Autodesk Fusion 360 part; units mm, degrees
(part 2 of 2)
  spline S235 degree 3 poles (6.52, 51.4668) (6.4718, 51.4632) (6.3612, 51.455) (6.2503, 51.4547) (6.1877, 51.4545) knots 0 0 0 0 0.014491 0.033263 0.033263 0.033263 0.033263
  spline S236 degree 3 poles (6.1877, 51.4545) (6.1361, 51.4547) (6.0447, 51.4549) (5.9536, 51.4611) (5.9138, 51.4637) knots 0 0 0 0 0.015463 0.027406 0.027406 0.027406 0.027406
  spline S237 degree 3 poles (5.9138, 51.4637) (5.8835, 51.4668) (5.8299, 51.4722) (5.7791, 51.4899) (5.7569, 51.4976) knots 0 0 0 0 0.009095 0.016102 0.016102 0.016102 0.016102
  spline S238 degree 3 poles (5.7569, 51.4976) (5.7399, 51.506) (5.7078, 51.5219) (5.6847, 51.5493) (5.6738, 51.5622) knots 0 0 0 0 0.00562 0.010625 0.010625 0.010625 0.010625
  spline S239 degree 3 poles (5.6738, 51.5622) (5.6645, 51.5771) (5.6442, 51.6095) (5.6295, 51.6447) (5.6215, 51.6637) knots 0 0 0 0 0.005277 0.011439 0.011439 0.011439 0.011439
  line L59 (5.6215, 51.6637) -> (3.3385, 58.3653)
  line L60 (3.3385, 58.3653) -> (3.3323, 58.3653)
  line L61 (3.3323, 58.3653) -> (1.1108, 51.676)
  spline S240 degree 3 poles (1.1108, 51.676) (1.1048, 51.6553) (1.0938, 51.617) (1.0759, 51.5815) (1.0677, 51.5653) knots 0 0 0 0 0.006471 0.011908 0.011908 0.011908 0.011908
  spline S241 degree 3 poles (1.0677, 51.5653) (1.0572, 51.5514) (1.0346, 51.5214) (1.0001, 51.5059) (0.9815, 51.4976) knots 0 0 0 0 0.005123 0.011115 0.011115 0.011115 0.011115
  spline S242 degree 3 poles (0.9815, 51.4976) (0.9571, 51.4899) (0.901, 51.4722) (0.8423, 51.4668) (0.8092, 51.4637) knots 0 0 0 0 0.007671 0.017604 0.017604 0.017604 0.017604
  spline S243 degree 3 poles (0.8092, 51.4637) (0.7662, 51.4611) (0.6678, 51.4549) (0.5693, 51.4547) (0.5138, 51.4545) knots 0 0 0 0 0.012942 0.029559 0.029559 0.029559 0.029559
  spline S244 degree 3 poles (0.5138, 51.4545) (0.4569, 51.4547) (0.3561, 51.4551) (0.2559, 51.4654) (0.2123, 51.4699) knots 0 0 0 0 0.017081 0.030209 0.030209 0.030209 0.030209
  spline S245 degree 3 poles (0.2123, 51.4699) (0.1801, 51.4746) (0.125, 51.4825) (0.0802, 51.5149) (0.0615, 51.5284) knots 0 0 0 0 0.009571 0.01638 0.01638 0.01638 0.01638
  spline S246 degree 3 poles (0.0615, 51.5284) (0.0504, 51.5455) (0.0257, 51.5837) (0.029, 51.6294) (0.0308, 51.6545) knots 0 0 0 0 0.005987 0.013301 0.013301 0.013301 0.013301
  spline S247 degree 3 poles (0.0308, 51.6545) (0.0364, 51.6868) (0.0494, 51.7613) (0.0748, 51.8325) (0.0892, 51.873) knots 0 0 0 0 0.009806 0.02265 0.02265 0.02265 0.02265
  line L62 (0.0892, 51.873) -> (2.6862, 59.2699)
  spline S248 degree 3 poles (-5.6769, 59.0176) (-5.6766, 59.0522) (-5.6759, 59.1171) (-5.6682, 59.1815) (-5.6646, 59.2114) knots 0 0 0 0 0.010389 0.019436 0.019436 0.019436 0.019436
  spline S249 degree 3 poles (-5.6646, 59.2114) (-5.6602, 59.2372) (-5.6518, 59.2853) (-5.6311, 59.3294) (-5.6215, 59.3499) knots 0 0 0 0 0.007801 0.014559 0.014559 0.014559 0.014559
  spline S250 degree 3 poles (-5.6215, 59.3499) (-5.6115, 59.3667) (-5.5929, 59.3978) (-5.5641, 59.4198) (-5.5508, 59.4299) knots 0 0 0 0 0.005804 0.010768 0.010768 0.010768 0.010768
  spline S251 degree 3 poles (-5.5508, 59.4299) (-5.537, 59.4371) (-5.509, 59.4516) (-5.4775, 59.4535) (-5.4615, 59.4545) knots 0 0 0 0 0.004616 0.009349 0.009349 0.009349 0.009349
  line L63 (-5.4615, 59.4545) -> (-1.64, 59.4545)
  spline S252 degree 3 poles (-1.64, 59.4545) (-1.5929, 59.4501) (-1.4957, 59.4409) (-1.4143, 59.3869) (-1.3723, 59.3591) knots 0 0 0 0 0.013974 0.028812 0.028812 0.028812 0.028812
  spline S253 degree 3 poles (-1.3723, 59.3591) (-1.3356, 59.3174) (-1.2523, 59.2225) (-1.2484, 59.0951) (-1.2462, 59.0237) knots 0 0 0 0 0.016203 0.03683 0.03683 0.03683 0.03683
  line L64 (-1.2462, 59.0237) -> (-1.2462, 51.9222)
  spline S254 degree 3 poles (-1.2462, 51.9222) (-1.2484, 51.8509) (-1.2523, 51.7235) (-1.3356, 51.6286) (-1.3723, 51.5868) knots 0 0 0 0 0.020627 0.03683 0.03683 0.03683 0.03683
  spline S255 degree 3 poles (-1.3723, 51.5868) (-1.4143, 51.559) (-1.4957, 51.505) (-1.5929, 51.4959) (-1.64, 51.4914) knots 0 0 0 0 0.014838 0.028813 0.028813 0.028813 0.028813
  line L65 (-1.64, 51.4914) -> (-5.4185, 51.4914)
  spline S256 degree 3 poles (-5.4185, 51.4914) (-5.4344, 51.4924) (-5.4659, 51.4943) (-5.4939, 51.5089) (-5.5077, 51.516) knots 0 0 0 0 0.004732 0.009349 0.009349 0.009349 0.009349
  spline S257 degree 3 poles (-5.5077, 51.516) (-5.5206, 51.5261) (-5.5484, 51.5476) (-5.564, 51.5792) (-5.5723, 51.596) knots 0 0 0 0 0.004849 0.010403 0.010403 0.010403 0.010403
  spline S258 degree 3 poles (-5.5723, 51.596) (-5.5803, 51.6167) (-5.5977, 51.6616) (-5.6072, 51.7089) (-5.6123, 51.7345) knots 0 0 0 0 0.006618 0.014436 0.014436 0.014436 0.014436
  spline S259 degree 3 poles (-5.6123, 51.7345) (-5.6168, 51.7655) (-5.6267, 51.8338) (-5.6273, 51.9029) (-5.6277, 51.9407) knots 0 0 0 0 0.009379 0.020693 0.020693 0.020693 0.020693
  spline S260 degree 3 poles (-5.6277, 51.9407) (-5.6272, 51.9753) (-5.6264, 52.0403) (-5.6168, 52.1046) (-5.6123, 52.1345) knots 0 0 0 0 0.010392 0.019465 0.019465 0.019465 0.019465
  spline S261 degree 3 poles (-5.6123, 52.1345) (-5.6073, 52.1599) (-5.598, 52.2063) (-5.5803, 52.2501) (-5.5723, 52.2699) knots 0 0 0 0 0.007743 0.014145 0.014145 0.014145 0.014145
  spline S262 degree 3 poles (-5.5723, 52.2699) (-5.5639, 52.2859) (-5.5479, 52.3163) (-5.5206, 52.337) (-5.5077, 52.3468) knots 0 0 0 0 0.005357 0.010155 0.010155 0.010155 0.010155
  spline S263 degree 3 poles (-5.5077, 52.3468) (-5.4939, 52.354) (-5.4659, 52.3685) (-5.4344, 52.3705) (-5.4185, 52.3714) knots 0 0 0 0 0.004616 0.009349 0.009349 0.009349 0.009349
  line L66 (-5.4185, 52.3714) -> (-2.3046, 52.3714)
  line L67 (-2.3046, 52.3714) -> (-2.3046, 54.8699)
  line L68 (-2.3046, 54.8699) -> (-4.9754, 54.8699)
  spline S264 degree 3 poles (-4.9754, 54.8699) (-4.9914, 54.871) (-5.0233, 54.8733) (-5.0509, 54.8895) (-5.0646, 54.8976) knots 0 0 0 0 0.004743 0.009456 0.009456 0.009456 0.009456
  spline S265 degree 3 poles (-5.0646, 54.8976) (-5.0776, 54.908) (-5.1046, 54.9297) (-5.1228, 54.9592) (-5.1323, 54.9745) knots 0 0 0 0 0.004957 0.010314 0.010314 0.010314 0.010314
  spline S266 degree 3 poles (-5.1323, 54.9745) (-5.1411, 54.9938) (-5.1607, 55.0369) (-5.1682, 55.0839) (-5.1723, 55.1099) knots 0 0 0 0 0.006314 0.014174 0.014174 0.014174 0.014174
  spline S267 degree 3 poles (-5.1723, 55.1099) (-5.1759, 55.1411) (-5.1836, 55.2086) (-5.1843, 55.2765) (-5.1846, 55.313) knots 0 0 0 0 0.00943 0.020357 0.020357 0.020357 0.020357
  spline S268 degree 3 poles (-5.1846, 55.313) (-5.1843, 55.3474) (-5.1837, 55.4112) (-5.1759, 55.4745) (-5.1723, 55.5037) knots 0 0 0 0 0.010312 0.01913 0.01913 0.01913 0.01913
  spline S269 degree 3 poles (-5.1723, 55.5037) (-5.1681, 55.5282) (-5.1603, 55.573) (-5.141, 55.6142) (-5.1323, 55.633) knots 0 0 0 0 0.007409 0.013581 0.013581 0.013581 0.013581
  spline S270 degree 3 poles (-5.1323, 55.633) (-5.123, 55.648) (-5.1054, 55.6764) (-5.0777, 55.695) (-5.0646, 55.7037) knots 0 0 0 0 0.005231 0.009893 0.009893 0.009893 0.009893
  spline S271 degree 3 poles (-5.0646, 55.7037) (-5.0507, 55.71) (-5.0224, 55.7229) (-4.9913, 55.7245) (-4.9754, 55.7253) knots 0 0 0 0 0.004529 0.009252 0.009252 0.009252 0.009252
  line L69 (-4.9754, 55.7253) -> (-2.3046, 55.7253)
  line L70 (-2.3046, 55.7253) -> (-2.3046, 58.5745)
  line L71 (-2.3046, 58.5745) -> (-5.4615, 58.5745)
  spline S272 degree 3 poles (-5.4615, 58.5745) (-5.4775, 58.5755) (-5.509, 58.5774) (-5.537, 58.5919) (-5.5508, 58.5991) knots 0 0 0 0 0.004732 0.009348 0.009348 0.009348 0.009348
  spline S273 degree 3 poles (-5.5508, 58.5991) (-5.564, 58.609) (-5.5924, 58.6302) (-5.6114, 58.6601) (-5.6215, 58.676) knots 0 0 0 0 0.004915 0.010531 0.010531 0.010531 0.010531
  spline S274 degree 3 poles (-5.6215, 58.676) (-5.6312, 58.6958) (-5.6521, 58.7387) (-5.6602, 58.7859) (-5.6646, 58.8114) knots 0 0 0 0 0.006545 0.014271 0.014271 0.014271 0.014271
  spline S275 degree 3 poles (-5.6646, 58.8114) (-5.6682, 58.8424) (-5.6761, 58.9109) (-5.6766, 58.9798) (-5.6769, 59.0176) knots 0 0 0 0 0.009353 0.020665 0.020665 0.020665 0.020665
  spline S276 degree 3 poles (-13.4185, 59.0176) (-13.4172, 59.056) (-13.4149, 59.1281) (-13.3892, 59.1954) (-13.3771, 59.2268) knots 0 0 0 0 0.011431 0.021461 0.021461 0.021461 0.021461
  spline S277 degree 3 poles (-13.3771, 59.2268) (-13.3626, 59.254) (-13.3342, 59.3071) (-13.2903, 59.3483) (-13.2689, 59.3684) knots 0 0 0 0 0.009183 0.01792 0.01792 0.01792 0.01792
  spline S278 degree 3 poles (-13.2689, 59.3684) (-13.246, 59.3855) (-13.2003, 59.4198) (-13.1463, 59.4389) (-13.1194, 59.4484) knots 0 0 0 0 0.008537 0.01705 0.01705 0.01705 0.01705
  spline S279 degree 3 poles (-13.1194, 59.4484) (-13.0919, 59.4555) (-13.0377, 59.4697) (-12.9816, 59.4719) (-12.9538, 59.473) knots 0 0 0 0 0.008479 0.016779 0.016779 0.016779 0.016779
  line L72 (-12.9538, 59.473) -> (-12.6038, 59.473)
  spline S280 degree 3 poles (-12.6038, 59.473) (-12.5519, 59.472) (-12.4542, 59.47) (-12.3589, 59.449) (-12.3142, 59.4391) knots 0 0 0 0 0.015537 0.029222 0.029222 0.029222 0.029222
  spline S281 degree 3 poles (-12.3142, 59.4391) (-12.2729, 59.4252) (-12.188, 59.3965) (-12.1158, 59.3433) (-12.0788, 59.316) knots 0 0 0 0 0.013 0.026713 0.026713 0.026713 0.026713
  spline S282 degree 3 poles (-12.0788, 59.316) (-12.0405, 59.282) (-11.958, 59.2086) (-11.8916, 59.1203) (-11.856, 59.073) knots 0 0 0 0 0.015332 0.033042 0.033042 0.033042 0.033042
  spline S283 degree 3 poles (-11.856, 59.073) (-11.8168, 59.0151) (-11.7307, 58.8882) (-11.6588, 58.7528) (-11.6196, 58.6791) knots 0 0 0 0 0.020961 0.045964 0.045964 0.045964 0.045964
  line L73 (-11.6196, 58.6791) -> (-9.1904, 54.1499)
  spline S284 degree 3 poles (-9.1904, 54.1499) (-9.1262, 54.0304) (-8.9953, 53.7868) (-8.8701, 53.5402) (-8.8064, 53.4145) knots 0 0 0 0 0.040696 0.082963 0.082963 0.082963 0.082963
  spline S285 degree 3 poles (-8.8064, 53.4145) (-8.7435, 53.2884) (-8.6202, 53.0407) (-8.5034, 52.7899) (-8.4462, 52.6668) knots 0 0 0 0 0.042275 0.082998 0.082998 0.082998 0.082998
  line L74 (-8.4462, 52.6668) -> (-8.4338, 52.6668)
  spline S286 degree 3 poles (-8.4338, 52.6668) (-8.4377, 52.816) (-8.4455, 53.1175) (-8.45, 53.4191) (-8.4523, 53.5714) knots 0 0 0 0 0.044782 0.090481 0.090481 0.090481 0.090481
  spline S287 degree 3 poles (-8.4523, 53.5714) (-8.4541, 53.7248) (-8.4577, 54.0304) (-8.4582, 54.336) (-8.4585, 54.4884) knots 0 0 0 0 0.046002 0.091695 0.091695 0.091695 0.091695
  line L75 (-8.4585, 54.4884) -> (-8.4585, 59.2945)
  spline S288 degree 3 poles (-8.4585, 59.2945) (-8.4573, 59.3089) (-8.4548, 59.3385) (-8.4401, 59.3643) (-8.4325, 59.3776) knots 0 0 0 0 0.00428 0.008798 0.008798 0.008798 0.008798
  spline S289 degree 3 poles (-8.4325, 59.3776) (-8.4216, 59.3904) (-8.3978, 59.4184) (-8.3635, 59.4318) (-8.3449, 59.4391) knots 0 0 0 0 0.004969 0.010857 0.010857 0.010857 0.010857
  spline S290 degree 3 poles (-8.3449, 59.4391) (-8.3212, 59.4463) (-8.2679, 59.4623) (-8.213, 59.4711) (-8.1825, 59.476) knots 0 0 0 0 0.007418 0.016666 0.016666 0.016666 0.016666
  spline S291 degree 3 poles (-8.1825, 59.476) (-8.1444, 59.4805) (-8.0592, 59.4905) (-7.9734, 59.4911) (-7.926, 59.4914) knots 0 0 0 0 0.011505 0.025717 0.025717 0.025717 0.025717
  spline S292 degree 3 poles (-7.926, 59.4914) (-7.8785, 59.4911) (-7.7928, 59.4905) (-7.7076, 59.4805) (-7.6695, 59.476) knots 0 0 0 0 0.014211 0.025712 0.025712 0.025712 0.025712
  spline S293 degree 3 poles (-7.6695, 59.476) (-7.6393, 59.4712) (-7.5853, 59.4626) (-7.5333, 59.4463) (-7.5104, 59.4391) knots 0 0 0 0 0.009166 0.01635 0.01635 0.01635 0.01635
  spline S294 degree 3 poles (-7.5104, 59.4391) (-7.4926, 59.4317) (-7.4595, 59.4179) (-7.4366, 59.3904) (-7.426, 59.3776) knots 0 0 0 0 0.005673 0.010586 0.010586 0.010586 0.010586
  spline S295 degree 3 poles (-7.426, 59.3776) (-7.4184, 59.3643) (-7.4037, 59.3385) (-7.4012, 59.3089) (-7.4, 59.2945) knots 0 0 0 0 0.004518 0.008798 0.008798 0.008798 0.008798
  line L76 (-7.4, 59.2945) -> (-7.4, 51.9468)
  spline S296 degree 3 poles (-7.4, 51.9468) (-7.4031, 51.8729) (-7.4088, 51.7385) (-7.4991, 51.6403) (-7.5398, 51.596) knots 0 0 0 0 0.021365 0.038854 0.038854 0.038854 0.038854
  spline S297 degree 3 poles (-7.5398, 51.596) (-7.587, 51.5655) (-7.68, 51.5054) (-7.7903, 51.496) (-7.8446, 51.4914) knots 0 0 0 0 0.016583 0.032673 0.032673 0.032673 0.032673
  line L77 (-7.8446, 51.4914) -> (-8.3655, 51.4914)
  spline S298 degree 3 poles (-8.3655, 51.4914) (-8.422, 51.4922) (-8.5256, 51.4935) (-8.6273, 51.5132) (-8.6735, 51.5222) knots 0 0 0 0 0.016925 0.031011 0.031011 0.031011 0.031011
  spline S299 degree 3 poles (-8.6735, 51.5222) (-8.7135, 51.534) (-8.7925, 51.5572) (-8.8617, 51.6018) (-8.8958, 51.6237) knots 0 0 0 0 0.012439 0.024552 0.024552 0.024552 0.024552
  spline S300 degree 3 poles (-8.8958, 51.6237) (-8.9292, 51.6508) (-9.0006, 51.7088) (-9.0566, 51.7818) (-9.0863, 51.8207) knots 0 0 0 0 0.01286 0.027486 0.027486 0.027486 0.027486
  spline S301 degree 3 poles (-9.0863, 51.8207) (-9.1186, 51.8676) (-9.1887, 51.9698) (-9.2477, 52.0787) (-9.2796, 52.1376) knots 0 0 0 0 0.017076 0.037143 0.037143 0.037143 0.037143
  line L78 (-9.2796, 52.1376) -> (-11.1471, 55.633)
  spline S302 degree 3 poles (-11.1471, 55.633) (-11.2037, 55.7383) (-11.3155, 55.9461) (-11.4258, 56.1547) (-11.4802, 56.2576) knots 0 0 0 0 0.035874 0.070788 0.070788 0.070788 0.070788
  spline S303 degree 3 poles (-11.4802, 56.2576) (-11.533, 56.3582) (-11.6375, 56.5575) (-11.7391, 56.7582) (-11.7895, 56.8576) knots 0 0 0 0 0.034092 0.067503 0.067503 0.067503 0.067503
  spline S304 degree 3 poles (-11.7895, 56.8576) (-11.8387, 56.9553) (-11.9365, 57.1493) (-12.035, 57.343) (-12.0838, 57.4391) knots 0 0 0 0 0.03283 0.06518 0.06518 0.06518 0.06518
  spline S305 degree 3 poles (-12.0838, 57.4391) (-12.1323, 57.5347) (-12.2294, 57.726) (-12.3246, 57.9183) (-12.3723, 58.0145) knots 0 0 0 0 0.032146 0.064365 0.064365 0.064365 0.064365
  line L79 (-12.3723, 58.0145) -> (-12.3785, 58.0145)
  spline S306 degree 3 poles (-12.3785, 58.0145) (-12.3747, 57.8491) (-12.3671, 57.5117) (-12.3644, 57.1743) (-12.3631, 57.0022) knots 0 0 0 0 0.049625 0.101244 0.101244 0.101244 0.101244
  spline S307 degree 3 poles (-12.3631, 57.0022) (-12.3622, 56.8302) (-12.3604, 56.4927) (-12.3601, 56.1553) (-12.36, 55.9899) knots 0 0 0 0 0.051616 0.101231 0.101231 0.101231 0.101231
  line L80 (-12.36, 55.9899) -> (-12.36, 51.6699)
  spline S308 degree 3 poles (-12.36, 51.6699) (-12.3611, 51.6557) (-12.3634, 51.627) (-12.3784, 51.6024) (-12.386, 51.5899) knots 0 0 0 0 0.004204 0.008515 0.008515 0.008515 0.008515
  spline S309 degree 3 poles (-12.386, 51.5899) (-12.397, 51.5776) (-12.4217, 51.5501) (-12.4551, 51.5341) (-12.4736, 51.5253) knots 0 0 0 0 0.004915 0.010984 0.010984 0.010984 0.010984
  spline S310 degree 3 poles (-12.4736, 51.5253) (-12.4972, 51.5165) (-12.5498, 51.4971) (-12.6053, 51.4895) (-12.636, 51.4853) knots 0 0 0 0 0.00753 0.016765 0.016765 0.016765 0.016765
  spline S311 degree 3 poles (-12.636, 51.4853) (-12.6746, 51.4817) (-12.7621, 51.4736) (-12.8499, 51.4732) (-12.8989, 51.473) knots 0 0 0 0 0.011645 0.026338 0.026338 0.026338 0.026338
  spline S312 degree 3 poles (-12.8989, 51.473) (-12.9434, 51.4733) (-13.0258, 51.4739) (-13.1079, 51.4817) (-13.1457, 51.4853) knots 0 0 0 0 0.013317 0.024719 0.024719 0.024719 0.024719
  spline S313 degree 3 poles (-13.1457, 51.4853) (-13.1769, 51.4893) (-13.2326, 51.4966) (-13.285, 51.5165) (-13.3081, 51.5253) knots 0 0 0 0 0.009394 0.016772 0.016772 0.016772 0.016772
  spline S314 degree 3 poles (-13.3081, 51.5253) (-13.3257, 51.5342) (-13.3579, 51.5505) (-13.3817, 51.5776) (-13.3925, 51.5899) knots 0 0 0 0 0.00586 0.010718 0.010718 0.010718 0.010718
  spline S315 degree 3 poles (-13.3925, 51.5899) (-13.4001, 51.6024) (-13.415, 51.627) (-13.4173, 51.6557) (-13.4185, 51.6699) knots 0 0 0 0 0.004311 0.008515 0.008515 0.008515 0.008515
  line L81 (-13.4185, 51.6699) -> (-13.4185, 59.0176)
  point P0 (0, 47.7622)
  point P1 (0, 47.7622)
  dimension "d26" = 2
  dimension "d27" = 1
  constraint coincident L1.end L2.start
  constraint coincident L6 L8.end
  constraint perpendicular L6 L8
  constraint coincident L0.end L1.start
  constraint coincident L4 L9.end
  constraint perpendicular L4 L9
  constraint midpoint A2 L10.end
  constraint midpoint A3 L11.end
  constraint coincident L10 P1
  constraint coincident L11 P1
  constraint horizontal L12
  constraint perpendicular L12 L13
  constraint parallel L12 L14
  constraint parallel L13 L15
  constraint coincident L16 P1
  constraint coincident L17 P1
  constraint coincident P1 P0
  measures "d26" distance of L13.end L14.end
  measures "d27" distance of L12.end L13.end
extrude "Extrude3" cut sketch "Sketch2" against normal blind 1 contours S0 S1 S2 S3 S4 S5 S6 S7 L18 S8 S9 S10 S11 L19 L20 S12 S13 S14 S15 S16 S17 S18 S19 L21 S20 S21 L22 S22 S23 S24 S25 S26 S27 S28 S29 S30 S31 S32 S33 S34 S35 L23 S36 S37 | S46 S47 S48 S49 L27 S50 S51 L28 S52 S53 L29 S54 S55 S56 S57 S58 S59 S60 S61 L30 L31 L32 S62 S63 S64 S65 S66 S67 S68 S69 L33 L34 L35 S70 S71 S72 S73 | S74 S75 S76 S77 L36 L37 L38 S78 S79 S80 S81 S82 S83 S84 S85 L39 L40 S86 S87 S88 S89 S90 S91 S92 S93 L41 S94 S95 L42 S96 S97 S98 S99 | S100 S101 S102 S103 L43 S104 S105 L44 S106 S107 S108 S109 S110 S111 S112 S113 L45 L46 S114 S115 S116 S117 | S118 S119 S120 S121 S122 S123 S124 S125 S126 S127 S128 S129 S130 S131 S132 S133 | S150 S151 S152 S153 S154 S155 S156 S157 L47 L48 L49 S158 S159 S160 S161 S162 S163 S164 S165 L50 S166 S167 S168 S169 S170 S171 S172 S173 L51 L52 L53 S174 S175 S176 S177 S178 S179 S180 S181 L54 L55 L56 S182 S183 S184 S185 S186 S187 S188 S189 L57 | S190 S191 S192 S193 S194 S195 S196 S197 S198 S199 S200 S201 S202 S203 S204 S205 | S222 S223 S224 S225 S226 S227 S228 S229 S230 S231 L58 S232 S233 S234 S235 S236 S237 S238 S239 L59 L60 L61 S240 S241 S242 S243 S244 S245 S246 S247 L62 | S248 S249 S250 S251 L63 S252 S253 L64 S254 S255 L65 S256 S257 S258 S259 S260 S261 S262 S263 L66 L67 L68 S264 S265 S266 S267 S268 S269 S270 S271 L69 L70 L71 S272 S273 S274 S275 | S276 S277 S278 S279 L72 S280 S281 S282 S283 L73 S284 S285 L74 S286 S287 L75 S288 S289 S290 S291 S292 S293 S294 S295 L76 S296 S297 L77 S298 S299 S300 S301 L78 S302 S303 S304 S305 L79 S306 S307 L80 S308 S309 S310 S311 S312 S313 S314 S315 L81
